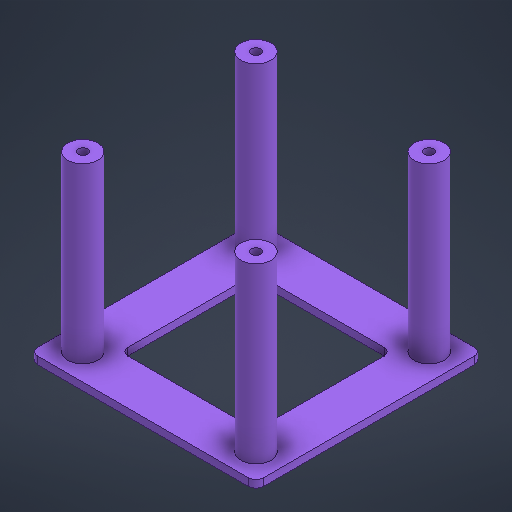
# Autodesk Inventor part: lidar base
Saved by Autodesk Inventor 2026 (Build 300175000, 175)
## iProperties
Created: 2025-04-15
Part Number: lidar base
Material: Generic
Document SubType Name: Modeling
Designer: ADM
Density: 1 g/cm^3
Appearance: Violet
Author: ADM
Autodesk Inventor part; units mm, degrees
ref_plane "YZ Plane" through (0, 0, 0) normal (1, 0, 0) x (0, 1, 0)
ref_plane "XZ Plane" through (0, 0, 0) normal (0, 1, 0) x (-1, 0, 0)
sketch "Sketch2" plane through (0, 0, 0) normal (0, 1, 0) x (-1, 0, 0)
  line L0 (2, 0) -> (58, 0)
  line L1 (60, -2) -> (60, -58)
  line L2 (58, -60) -> (2, -60)
  line L3 (0, -58) -> (0, -2)
  line L4 (48, -46) -> (48, -14)
  line L5 (46, -12) -> (14, -12)
  line L6 (12, -14) -> (12, -46)
  line L7 (14, -48) -> (46, -48)
  arc A0 (60, -2) -> (58, 0) centre (58, -2) ccw
  arc A1 (58, -60) -> (60, -58) centre (58, -58) ccw
  arc A2 (0, -58) -> (2, -60) centre (2, -58) ccw
  arc A3 (2, 0) -> (0, -2) centre (2, -2) ccw
  arc A4 (14, -12) -> (12, -14) centre (14, -14) ccw
  arc A5 (12, -46) -> (14, -48) centre (14, -46) ccw
  arc A6 (46, -48) -> (48, -46) centre (46, -46) ccw
  arc A7 (48, -14) -> (46, -12) centre (46, -14) ccw
  point P0 (0, 0)
  point P1 (60, -60)
  point P2 (60, 0)
  point P3 (0, -60)
  dimension "d9" = 60
  dimension "d10" = 60
  dimension "d11" = 12
  dimension "d12" = 2
  constraints: 16 end point, 16 point on circle, 16 tangent, 8 centre point, 8 point on line, 7 equal radius, 4 parallel, 2 perpendicular, 1 horizontal, 3 other
  measures "d9" distance of point (60, -60) point (0, -60)
  measures "d10" distance of point (60, 0) point (60, -60)
  measures "d11" distance between parallel lines of L1 L4
  measures "d12" radius of A0
extrude "Extrusion2" add sketch "Sketch2" along normal blind 2
sketch "Sketch3" plane through (0, 2, 0) normal (0, 1, 0) x (1, 0, 0)
  circle A0 centre (-53, 7) radius 4
  circle A1 centre (-7, 7) radius 4
  circle A2 centre (-53, 53) radius 4
  circle A3 centre (-7, 53) radius 4
  line L0 (-58, 0) -> (-2, 0) projected
  line L1 (-60, 58) -> (-60, 2) projected
  line L2 (-2, 60) -> (-58, 60) projected
  line L3 (0, 2) -> (0, 58) projected
  point P0 (0, 0)
  dimension "d15" = 8
  dimension "d16" = 8
  dimension "d17" = 8
  dimension "d18" = 8
  dimension "d19" = 7
  dimension "d20" = 7
  dimension "d21" = 7
  dimension "d22" = 7
  dimension "d23" = 7
  dimension "d24" = 7
  dimension "d25" = 7
  dimension "d26" = 7
  constraints: 4 centre point
  measures "d15" diameter of A0
  measures "d16" diameter of A1
  measures "d17" diameter of A2
  measures "d18" diameter of A3
  measures "d19" distance from line of L0 A0.centre
  measures "d20" distance from line of L1 A0.centre
  measures "d21" distance from line of L1 A2.centre
  measures "d22" distance from line of L2 A2.centre
  measures "d23" distance from line of L0 A1.centre
  measures "d24" distance from line of L3 A1.centre
  measures "d25" distance from line of L3 A3.centre
  measures "d26" distance from line of L2 A3.centre
extrude "Extrusion4" add sketch "Sketch3" along normal blind 46
ref_plane "Work Plane1" through (-7, 48, -53) normal (0, 1, 0) x (1, 0, 0)
sketch "Sketch5" plane through (-7, 48, -53) normal (0, 1, 0) x (1, 0, 0)
  circle A0 centre (-46, 0) radius 4 projected
  circle A1 centre (-46, 0) radius 1.25
  circle A2 centre (0, 0) radius 4 projected
  circle A3 centre (0, 0) radius 1.25
  circle A4 centre (0, -46) radius 4 projected
  circle A5 centre (0, -46) radius 1.25
  circle A6 centre (-46, -46) radius 4 projected
  circle A7 centre (-46, -46) radius 1.25
  point P0 (7, -53)
  dimension "d36" = 2.5
  dimension "d37" = 2.5
  dimension "d38" = 2.5
  dimension "d39" = 2.5
  constraints: 4 centre point, 4 coincident
  measures "d36" diameter of A1
  measures "d37" diameter of A3
  measures "d38" diameter of A5
  measures "d39" diameter of A7
extrude "Extrusion5" cut sketch "Sketch5" against normal blind 5 contours A1 | A3 | A5 | A7
body "Solid2"
